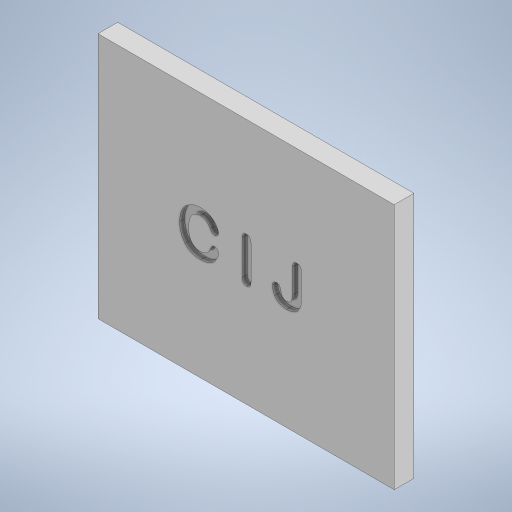
# Autodesk Inventor part: CIJ
Saved by Autodesk Inventor 2023 (Build 270158000, 158)
## iProperties
Created: 2022-08-29
Part Number: CIJ
Material: Genérico
Document SubType Name: Modeling
Designer: carlo
Density: 1 g/cm^3
Appearance: Valor por defecto
Author: carlo
Autodesk Inventor part; units mm, degrees
ref_plane "YZ Plane" through (0, 0, 0) normal (1, 0, 0) x (0, 1, 0)
ref_plane "XZ Plane" through (0, 0, 0) normal (0, 1, 0) x (-1, 0, 0)
ref_plane "XY Plane" through (0, 0, 0) normal (0, 0, 1) x (1, 0, 0)
sketch "Boceto1" plane through (0, 0, 0) normal (0, 0, 1) x (1, 0, 0)
  line L0 (0, 0) -> (300, 0)
  line L1 (300, 0) -> (300, 250)
  line L2 (300, 250) -> (0, 250)
  line L3 (0, 250) -> (0, 0)
  dimension "d0" = 300
  dimension "d1" = 250
  constraints: 8 end point, 2 parallel, 1 horizontal, 1 perpendicular
  measures "d0" distance of L1.end L2.end
  measures "d1" distance of L0.end L1.end
extrude "Extrusión1" add sketch "Boceto1" along normal blind 20
sketch "Boceto2" plane through (0, 0, 20) normal (0, 0, 1) x (1, 0, 0)
  line L0 (79.6353, 149.4956) -> (210.9697, 149.4956) construction
  line L1 (210.9697, 149.4956) -> (210.9697, 103.7275) construction
  line L2 (210.9697, 103.7275) -> (79.6353, 103.7275) construction
  line L3 (79.6353, 103.7275) -> (79.6353, 149.4956) construction
  spline S0 degree 2 poles (122.1217, 118.4599) (122.1217, 116.3303) (120.062, 111.4428) (115.5934, 106.695) (108.6462, 103.7275) (104.0379, 103.7275) knots 0 0 0 1 2 3 4 4 4
  spline S1 degree 2 poles (104.0379, 103.7275) (100.5469, 103.7275) (94.7866, 105.0541) (90.1085, 107.847) (88.1535, 110.1511) knots 0 0 0 1 2 3 3 3
  spline S2 degree 2 poles (88.1535, 110.1511) (86.408, 112.2458) (83.9293, 117.4126) (82.7075, 123.2427) (82.7075, 126.5592) knots 0 0 0 1 2 3 3 3
  spline S3 degree 2 poles (82.7075, 126.5592) (82.7075, 131.9005) (85.8145, 140.349) (91.6097, 146.3536) (99.3948, 149.4956) (103.7936, 149.4956) knots 0 0 0 1 2 3 4 4 4
  spline S4 degree 2 poles (103.7936, 149.4956) (109.1698, 149.4956) (117.5484, 145.2015) (122.017, 138.8827) (122.017, 136.0898) knots 0 0 0 1 2 3 3 3
  spline S5 degree 2 poles (122.017, 136.0898) (122.017, 134.5538) (119.8525, 132.2147) (118.3165, 132.2147) knots 0 0 0 1 2 2 2
  spline S6 degree 2 poles (118.3165, 132.2147) (116.5709, 132.2147) (114.8603, 133.8206) (113.813, 135.8105) knots 0 0 0 1 2 2 2
  spline S7 degree 2 poles (113.813, 135.8105) (112.0674, 139.1271) (107.3196, 142.3738) (103.8634, 142.3738) knots 0 0 0 1 2 2 2
  spline S8 degree 2 poles (103.8634, 142.3738) (98.3475, 142.3738) (91.7843, 133.9952) (91.7843, 126.245) knots 0 0 0 1 2 2 2
  spline S9 degree 2 poles (91.7843, 126.245) (91.7843, 121.0782) (94.6819, 114.2357) (99.9883, 110.8493) (103.5492, 110.8493) knots 0 0 0 1 2 3 3 3
  spline S10 degree 2 poles (103.5492, 110.8493) (107.4243, 110.8493) (112.7656, 114.6895) (114.1272, 118.3901) knots 0 0 0 1 2 2 2
  spline S11 degree 2 poles (114.1272, 118.3901) (114.6857, 120.1356) (116.3615, 122.3699) (118.2466, 122.3699) knots 0 0 0 1 2 2 2
  spline S12 degree 2 poles (118.2466, 122.3699) (119.8525, 122.3699) (122.1217, 120.1356) (122.1217, 118.4599) knots 0 0 0 1 2 2 2
  line L4 (146.0007, 109.2085) -> (146.0007, 144.0495)
  spline S13 degree 2 poles (146.0007, 144.0495) (146.0007, 146.7725) (148.4794, 149.4956) (150.4344, 149.4956) knots 0 0 0 1 2 2 2
  spline S14 degree 2 poles (150.4344, 149.4956) (152.4243, 149.4956) (154.9379, 146.8074) (154.9379, 144.0495) knots 0 0 0 1 2 2 2
  line L5 (154.9379, 144.0495) -> (154.9379, 109.2085)
  spline S15 degree 2 poles (154.9379, 109.2085) (154.9379, 106.4506) (152.4243, 103.7275) (150.4344, 103.7275) knots 0 0 0 1 2 2 2
  spline S16 degree 2 poles (150.4344, 103.7275) (148.5143, 103.7275) (146.0007, 106.4855) (146.0007, 109.2085) knots 0 0 0 1 2 2 2
  line L6 (206.0822, 144.0495) -> (206.0822, 120.8687)
  spline S17 degree 2 poles (206.0822, 120.8687) (206.0822, 117.8664) (205.5585, 113.6422) (204.6508, 111.4428) knots 0 0 0 1 2 2 2
  spline S18 degree 2 poles (204.6508, 111.4428) (203.1497, 107.8121) (196.2373, 103.7275) (191.2451, 103.7275) knots 0 0 0 1 2 2 2
  spline S19 degree 2 poles (191.2451, 103.7275) (186.7765, 103.7275) (180.7718, 106.5553) (178.9216, 109.7322) knots 0 0 0 1 2 2 2
  spline S20 degree 2 poles (178.9216, 109.7322) (177.9441, 111.4079) (176.7571, 115.8416) (176.7571, 117.8315) knots 0 0 0 1 2 2 2
  spline S21 degree 2 poles (176.7571, 117.8315) (176.7571, 119.9261) (179.0961, 122.1604) (180.9464, 122.1604) knots 0 0 0 1 2 2 2
  spline S22 degree 2 poles (180.9464, 122.1604) (182.7269, 122.1604) (184.5422, 120.1007) (185.031, 117.9362) knots 0 0 0 1 2 2 2
  spline S23 degree 2 poles (185.031, 117.9362) (185.5197, 115.6321) (186.567, 112.8393) (188.9759, 110.8493) (191.2102, 110.8493) knots 0 0 0 1 2 3 3 3
  spline S24 degree 2 poles (191.2102, 110.8493) (197.145, 110.8493) (197.145, 119.577) knots 0 0 0 1 1 1
  line L7 (197.145, 119.577) -> (197.145, 144.0495)
  spline S25 degree 2 poles (197.145, 144.0495) (197.145, 146.7725) (199.5189, 149.4956) (201.5787, 149.4956) knots 0 0 0 1 2 2 2
  spline S26 degree 2 poles (201.5787, 149.4956) (203.6384, 149.4956) (206.0822, 146.7725) (206.0822, 144.0495) knots 0 0 0 1 2 2 2
  point P0 (0, 0)
  constraints: 2 other
extrude "Extrusión2" cut sketch "Boceto2" against normal blind 5
